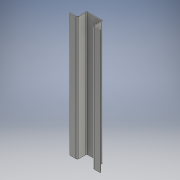
# Autodesk Inventor part: Reforço Bandeja
Saved by Autodesk Inventor 2017 (Build 210142000, 142)
## iProperties
Created: 2019-06-18
Part Number: Reforço Bandeja
Material: Stainless Steel AISI 304
Document SubType Name: Sheet Metal
Designer: leonardo.prado
Density: 8 g/cm^3
Sheet Metal Rule: Default_mm
Appearance: Chrome - Satin
Description: Chapa de Aço Inox Aisi 304 - #1,5mm
Mass: 273.823 g
Surface Area: 466.516 cm^2
Volume: 34.2279 cm^3
Flat Pattern Width: 9.25717 cm
Flat Pattern Length: 24.5 cm
Flat Pattern Area: 226.801 cm^2
Sheet Metal Width: 92,572 mm
Sheet Metal Length: 245,000 mm
Sheet Metal Area: 22680,062 mm^2
Author: leonardo.prado
Comments: 92 x 245
Autodesk Inventor part; units mm, degrees
note: some values were not read from the file. Chosen so that the rebuilt part matches the saved one: flange form of "Plate1".
ref_plane "YZ Plane" through (0, 0, 0) normal (1, 0, 0) x (0, 1, 0)
ref_plane "XZ Plane" through (0, 0, 0) normal (0, 1, 0) x (-1, 0, 0)
ref_plane "XY Plane" through (0, 0, 0) normal (0, 0, 1) x (1, 0, 0)
sketch "Sketch1" plane through (0, 0, 0) normal (0, 0, 1) x (1, 0, 0)
  line L0 (-15, 18.5) -> (15, 18.5)
  line L1 (-15, 18.5) -> (-15, 0)
  line L2 (15, 18.5) -> (15, 0)
  line L3 (-30, 0) -> (-15, 0)
  line L4 (15, 0) -> (30, 0)
  point P0 (0, 0)
  dimension "d0" = 30
  dimension "d1" = 15
  dimension "d3" = 18.5
  dimension "d4" = 15
  dimension "d5" = 15
  measures "d0" distance of L0.start L0.end
  measures "d1" distance from line of point (0, 0) L1
  measures "d3" distance from line of L0 point (0, 0)
  measures "d4" distance of L2.end L4.end
  measures "d5" distance of L3.start L1.end
contour flange "Contour Flange1" sketch "Sketch1" thickness 1.5 bend radius 1.5 width 245 along (0, 0, 1) mid plane yes both sides no wall seen from (-22.5, 0, 0) lies toward (0, 1, 0) curves L3 L1 L0 L2 L4
bend "Bend1"
corner "Corner1"
equation "\"d6\" = BendReliefWidth"
equation "\"d7\" = BendReliefDepth"
equation "\"d8\" = MinimumRemnant"
equation "\"d9\" = BendRadius"
equation "\"d11\" = BendRadius"
equation "\"d13\" = CornerReliefSize"
equation "\"d14\" = GapSize"
equation "\"d15\" = JacobiRadiusSize"
equation "\"d1\" = 0.5 * d0"
equation "\"BendRadius\" = Thickness"
equation "\"BendReliefWidth\" = Thickness"
equation "\"BendReliefDepth\" = 0.5 * Thickness"
equation "\"CornerReliefSize\" = 4 * Thickness"
equation "\"MinimumRemnant\" = 2 * Thickness"
equation "\"TransitionRadius\" = BendRadius"
equation "\"JacobiRadiusSize\" = BendRadius"
equation "\"GapSize\" = Thickness"
equation "\"Thickness\" = 1.5"
body "Solid1"
